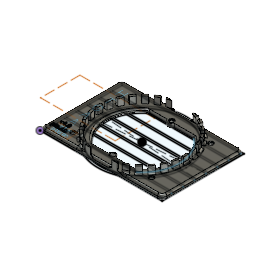
petriDishHolderRibsAndClaw (Autodesk Fusion 360 design; units mm, degrees)
Autodesk Fusion 360 part; units mm, degrees
sketch "main" plane through (0, 0, 0) normal (0, 0, 1) x (1, 0, 0)
  line L0 (0, 0) -> (127.76, 0)
  line L1 (127.76, 0) -> (127.76, 85.57)
  line L2 (127.76, 85.57) -> (0, 85.57)
  line L3 (0, 85.57) -> (0, 0)
  circle A0 centre (63.88, 42.785) radius 43.6
  circle A1 centre (63.88, 42.785) radius 46.2
  line L4 (-29.3174, 29.9498) -> (48.6581, 29.9498) construction
  line L5 (48.6581, 29.9498) -> (48.6581, 71.0126) construction
  line L6 (48.6581, 71.0126) -> (-29.3174, 71.0126) construction
  line L7 (-29.3174, 71.0126) -> (-29.3174, 29.9498) construction
  line L8 (2, 6.3389) -> (22.2506, 6.3389) construction
  line L9 (22.2506, 6.3389) -> (22.2506, 17.2311) construction
  line L10 (22.2506, 17.2311) -> (2, 17.2311) construction
  line L11 (2, 17.2311) -> (2, 6.3389) construction
  line L12 (41.8836, 72.785) -> (88.3277, 72.785)
  line L13 (41.8836, 12.785) -> (88.3277, 12.785)
  arc A2 (41.8836, 72.785) -> (41.8836, 12.785) centre (63.88, 42.785) ccw
  arc A3 (88.3277, 12.785) -> (88.3277, 72.785) centre (63.88, 42.785) ccw
  circle A4 centre (63.88, 42.785) radius 43.2
  line L14 (2, 47.785) -> (125.7601, 47.785)
  line L15 (125.76, 47.785) -> (125.76, 37.785)
  line L16 (125.76, 37.785) -> (2, 37.785)
  line L17 (2, 37.785) -> (2, 47.785)
  line L18 (2, 47.785) -> (125.76, 37.785) construction
  line L19 (125.76, 47.785) -> (2, 37.785) construction
  line L20 (125.7601, 47.785) -> (125.76, 47.785)
  line L21 (2, 11.785) -> (125.7601, 11.785)
  line L22 (2, 1.785) -> (2, 11.785)
  line L23 (125.76, 1.785) -> (2, 1.785)
  line L24 (125.76, 11.785) -> (125.76, 1.785)
  line L25 (125.7601, 11.785) -> (125.76, 11.785)
  line L26 (2, 23.785) -> (125.7601, 23.785)
  line L27 (2, 13.785) -> (2, 23.785)
  line L28 (125.76, 13.785) -> (2, 13.785)
  line L29 (125.76, 23.785) -> (125.76, 13.785)
  line L30 (125.7601, 23.785) -> (125.76, 23.785)
  line L31 (2, 35.785) -> (125.7601, 35.785)
  line L32 (2, 25.785) -> (2, 35.785)
  line L33 (125.76, 25.785) -> (2, 25.785)
  line L34 (125.76, 35.785) -> (125.76, 25.785)
  line L35 (125.7601, 35.785) -> (125.76, 35.785)
  line L36 (2, 59.785) -> (125.7601, 59.785)
  line L37 (2, 49.785) -> (2, 59.785)
  line L38 (125.76, 49.785) -> (2, 49.785)
  line L39 (125.76, 59.785) -> (125.76, 49.785)
  line L40 (125.7601, 59.785) -> (125.76, 59.785)
  line L41 (2, 71.785) -> (125.7601, 71.785)
  line L42 (2, 61.785) -> (2, 71.785)
  line L43 (125.76, 61.785) -> (2, 61.785)
  line L44 (125.76, 71.785) -> (125.76, 61.785)
  line L45 (125.7601, 71.785) -> (125.76, 71.785)
  line L46 (2, 83.785) -> (125.7601, 83.785)
  line L47 (2, 73.785) -> (2, 83.785)
  line L48 (125.76, 73.785) -> (2, 73.785)
  line L49 (125.76, 83.785) -> (125.76, 73.785)
  line L50 (125.7601, 83.785) -> (125.76, 83.785)
  point P0 (63.88, 42.785)
  dimension "d4" = 127.76
  dimension "d5" = 85.57
  dimension "d6" = 87.2
  dimension "d10" = 63.88
  dimension "d11" = 42.785
  dimension "d12" = 92.4
  dimension "d39" = 74.4
  dimension "d42" = 8
  dimension "d61" = 4
  dimension "d67" = 30
  dimension "d68" = 30
  dimension "d72" = 86.4
  dimension "d78" = 10
  dimension "d81" = 0
  dimension "d82" = 12
  dimension "d86" = 2
  dimension "d87" = 5
  text T0 "v1.6\nplastic" font "Arial" height 4 align centre middle in box 20.2506 x 10.8923 at (2, 6.3389) x (1, 0) y (0, 1) spacing 1 kerned
  constraint horizontal L0
  constraint vertical L1
  constraint horizontal L2
  constraint vertical L3
  constraint coincident L0.start L3.end
  constraint concentric A0 A1
  constraint concentric A0 A2
  constraint horizontal L12
  constraint horizontal L13
  constraint concentric A2 A3
  constraint coincident L12.end A3.end
  constraint coincident L12.start A2.start
  constraint concentric A3 A4
  constraint horizontal L14
  constraint perpendicular L14 L15
  constraint parallel L14 L16
  constraint parallel L15 L17
  constraint coincident L18 P0
  constraint coincident L19 P0
  constraint coincident P0 A0.centre
  constraint coincident L21.start
  constraint coincident L21
  measures "d4" distance of L0.start L0.end
  measures "d5" distance of L0.start L2.end
  measures "d6" diameter of A0
  measures "d10" horizontal distance of L0.start A0.centre
  measures "d11" vertical distance of L0.start A0.centre
  measures "d12" diameter of A1
  measures "d39" diameter of A2
  measures "d67" distance of P0 L12
  measures "d68" distance of P0 L13
  measures "d72" diameter of A4
  measures "d78" distance of L14.start L16.end
  measures "d86" distance of L1 L15
  measures "d87" distance of P0 L14
extrude "Extrude1" add sketch "main" along normal blind 4 contours L0 L2 L3 A1 L14 L16 L17 L21 L22 L23 L26 L27 L28 L31 L32 L33 L36 L37 L38 L41 L42 L43 L46 L47 L48 | L0 A0 A1 L23 | L0 A0 A4 L23 | A1 L21 L22 L23 | A0 A1 L21 L23 | L0 L1 L2 A1 L14 L15 L16 L21 L23 L24 L26 L28 L29 L31 L33 L34 L36 L38 L39 L41 L43 L44 L46 L48 L49 | L0 A0 A1 L23 | L2 A0 A1 L46 | L0 A4 L23 | A0 A4 L21 L23 | L0 A0 A4 L23 | A0 A1 L21 L28 | A0 A1 L21 L23 | A1 L21 L23 L24 | L2 A0 A4 L46 | L2 A0 A1 L46 | A0 A1 L46 L48 | A1 L46 L47 L48 | A4 L21 L23 | A0 A4 L21 L28 | A0 A4 L21 L23 | A1 L26 L27 L28 | A0 A1 L26 L28 | A0 A1 L21 L28 | L2 A4 L46 | L2 A0 A4 L46 | A0 A4 L46 L48 | A1 L46 L48 L49 | A0 A1 L46 L48 | A0 A1 L41 L48 | L13 A2 A3 A4 L21 L28 | A0 A4 L26 L28 | A0 A4 L21 L28 | A0 A1 L26 L33 | A0 A1 L26 L28 | A1 L26 L28 L29 | A4 L46 L48 | A0 A4 L46 L48 | A0 A4 L41 L48 | A0 A1 L41 L48 | A0 A1 L41 L43 | A1 L41 L42 L43 | A2 A4 L26 L28 | A0 A4 L26 L33 | A0 A4 L26 L28 | A1 L31 L32 L33 | A0 A1 L31 L33 | A0 A1 L26 L33 | L12 A2 A3 A4 L41 L48 | A0 A4 L41 L48 | A0 A4 L41 L43 | A1 L41 L43 L44 | A0 A1 L41 L43 | A0 A1 L36 L43 | A3 A4 L26 L28 | A2 A4 L26 L33 | L13 A2 A3 L28 | A2 A3 L26 L28 | A0 A4 L31 L33 | A0 A4 L26 L33 | A0 A1 L16 L31 | A0 A1 L31 L33 | A1 L31 L33 L34 | A2 A4 L41 L43 | A0 A4 L41 L43 | A0 A4 L36 L43 | A0 A1 L36 L43 | A0 A1 L36 L38 | A1 L36 L37 L38 | A3 A4 L26 L33 | A2 A4 L31 L33 | A2 A3 L26 L33 | A0 A4 L16 L31 | A0 A4 L31 L33 | A1 L14 L16 L17 | A0 A1 L14 L16 | A0 A1 L16 L31 | A3 A4 L41 L43 | A2 A4 L36 L43 | A2 A3 L41 L43 | L12 A2 A3 L41 | A0 A4 L36 L43 | A0 A4 L36 L38 | A1 L36 L38 L39 | A0 A1 L36 L38 | A0 A1 L14 L38 | A3 A4 L31 L33 | A2 A4 L16 L31 | A2 A3 L31 L33 | A0 A4 L14 L16 | A0 A4 L16 L31 | A0 A1 L14 L16 | A1 L14 L15 L16 | A3 A4 L36 L43 | A2 A4 L36 L38 | A2 A3 L36 L43 | A0 A4 L36 L38 | A0 A4 L14 L38 | A0 A1 L14 L38 | A3 A4 L16 L31 | A2 A4 L14 L16 | A2 A3 L16 L31 | A0 A4 L14 L16 | A3 A4 L36 L38 | A2 A4 L14 L38 | A2 A3 L36 L38 | A0 A4 L14 L38 | A3 A4 L14 L16 | A2 A3 L14 L16 | A3 A4 L14 L38 | A2 A3 L14 L38 makes body 1
extrude "Extrude2" add sketch "main" along normal blind 7 from surface at 4 contours L0 A0 A1 L23 | A0 A1 L21 L23 | L0 A0 A1 L23 | L2 A0 A1 L46 | A0 A1 L21 L28 | A0 A1 L21 L23 | L2 A0 A1 L46 | A0 A1 L46 L48 | A0 A1 L26 L28 | A0 A1 L21 L28 | A0 A1 L46 L48 | A0 A1 L41 L48 | A0 A1 L26 L33 | A0 A1 L26 L28 | A0 A1 L41 L48 | A0 A1 L41 L43 | A0 A1 L31 L33 | A0 A1 L26 L33 | A0 A1 L41 L43 | A0 A1 L36 L43 | A0 A1 L16 L31 | A0 A1 L31 L33 | A0 A1 L36 L43 | A0 A1 L36 L38 | A0 A1 L14 L16 | A0 A1 L16 L31 | A0 A1 L36 L38 | A0 A1 L14 L38 | A0 A1 L14 L16 | A0 A1 L14 L38 bodies 1
extrude "Extrude6" add sketch "main" along normal blind 2 from surface at 9 contours L0 A0 A4 L23 | A0 A4 L21 L23 | L2 A0 A4 L46 | A0 A4 L21 L28 | A0 A4 L46 L48 | A0 A4 L26 L28 | A0 A4 L41 L48 | A0 A4 L26 L33 | A0 A4 L41 L43 | A0 A4 L31 L33 | A0 A4 L36 L43 | A0 A4 L16 L31 | A0 A4 L36 L38 | A0 A4 L14 L16 | A0 A4 L14 L38 picked at (76.3561, 1.3005) picked at (79.8883, 2.6163) picked at (76.3561, 84.2695) picked at (94.3772, 12.0026) picked at (79.8883, 82.9537) picked at (96.9347, 14.824) picked at (94.3772, 73.5674) picked at (102.9314, 24.0055) picked at (96.9347, 70.746) picked at (104.1525, 26.8688) picked at (102.9314, 61.5645) picked at (106.6788, 36.0067) picked at (104.1525, 58.7012) picked at (106.9776, 47.2308) picked at (106.6788, 49.5633) bodies 1
fillet "Fillet9" radius 1 1 edges at (107.08, 42.785, 9) on bodies 1
fillet "Fillet9" radius 1 1 edges at (107.08, 42.785, 11) on bodies 1
fillet "Fillet4" radius 2 2 edges at (17.68, 42.785, 4) (110.08, 42.785, 4) on bodies 1
fillet "Fillet5" radius 2 13 edges at (0, 42.785, 4) (63.88, 85.57, 4) (106.9182, 85.57, 4) (83.3417, 85.57, 4.3962) (81.3123, 85.57, 8.5) (127.76, 42.785, 4) (81.3123, 0, 8.5) (83.3417, 0, 4.3962) (106.9182, 0, 4) (63.88, 0, 4) (20.8418, 0, 4) (44.4183, 0, 4.3962) (46.4477, 0, 8.5) on bodies 1
fillet "Fillet5" radius 2 3 edges at (46.4477, 85.57, 8.5) (44.4183, 85.57, 4.3962) (20.8418, 85.57, 4) on bodies 1
fillet "corners" radius 5 2 edges at (0, 0, 1) (0.5858, 0.5858, 3.4142) on bodies 1
fillet "corners" radius 5 2 edges at (127.76, 85.57, 1) (127.1742, 84.9842, 3.4142) on bodies 1
fillet "corners" radius 5 2 edges at (0.5858, 84.9842, 3.4142) (0, 85.57, 1) on bodies 1
fillet "corners" radius 5 2 edges at (127.76, 0, 1) (127.1742, 0.5858, 3.4142) on bodies 1
extrude "Extrude3" cut sketch "main" along normal blind 4 contours L13 A2 A3 L28 | A2 A3 L26 L28 | A2 A3 L26 L33 | A2 A3 L41 L43 | L12 A2 A3 L41 | A2 A3 L31 L33 | A2 A3 L36 L43 | A2 A3 L16 L31 | A2 A3 L36 L38 | A2 A3 L14 L16 | A2 A3 L14 L38 bodies 1
extrude "Extrude5" add sketch "main" along normal blind 1 from surface at 4 text T0 bodies 1
chamfer "Chamfer3" distance 1.5 angle 45 3 edges at (26.68, 42.785, 4) (102.58, 42.785, 4) (65.1057, 12.785, 4) tangent chain off on bodies 1
extrude "Extrude7" cut sketch "main" along normal blind 1 contours A1 L21 L22 L23 | A0 A1 L21 L23 | A0 A4 L21 L23 | A0 A1 L21 L23 | A1 L21 L23 L24 | L2 A0 A4 L46 | A0 A1 L46 L48 | A1 L46 L47 L48 | A4 L21 L23 | A0 A4 L21 L23 | A1 L26 L27 L28 | A0 A1 L26 L28 | L2 A0 A4 L46 | A0 A4 L46 L48 | A1 L46 L48 L49 | A0 A1 L46 L48 | A0 A1 L41 L48 | A0 A4 L26 L28 | A0 A1 L26 L33 | A0 A1 L26 L28 | A1 L26 L28 L29 | A4 L46 L48 | A0 A4 L46 L48 | A0 A1 L41 L48 | A0 A1 L41 L43 | A1 L41 L42 L43 | A2 A4 L26 L28 | A0 A4 L26 L28 | A1 L31 L32 L33 | A0 A1 L31 L33 | A0 A1 L26 L33 | A1 L41 L43 L44 | A0 A1 L41 L43 | A0 A1 L36 L43 | A3 A4 L26 L28 | A2 A3 L26 L28 | A0 A4 L31 L33 | A0 A1 L16 L31 | A0 A1 L31 L33 | A1 L31 L33 L34 | A2 A4 L41 L43 | A0 A1 L36 L43 | A0 A1 L36 L38 | A1 L36 L37 L38 | A2 A4 L31 L33 | A0 A4 L31 L33 | A1 L14 L16 L17 | A0 A1 L14 L16 | A0 A1 L16 L31 | A0 A4 L36 L38 | A1 L36 L38 L39 | A0 A1 L36 L38 | A0 A1 L14 L38 | A3 A4 L31 L33 | A2 A3 L31 L33 | A0 A4 L14 L16 | A0 A1 L14 L16 | A1 L14 L15 L16 | A2 A4 L36 L38 | A0 A4 L36 L38 | A0 A1 L14 L38 | A2 A4 L14 L16 | A0 A4 L14 L16 | A3 A4 L36 L38 | A2 A3 L36 L38 | A3 A4 L14 L16 | A2 A3 L14 L16 bodies 1
sketch "fingers" plane through (0, 0, 0) normal (0, 0, 1) x (1, 0, 0)
  line L0 (65.88, -8.3696) -> (61.88, -8.3696)
  line L1 (61.88, -8.3696) -> (61.88, 93.9396)
  line L2 (61.88, 93.9396) -> (65.88, 93.9396)
  line L3 (65.88, 93.9396) -> (65.88, -8.3696)
  line L4 (65.88, -8.3696) -> (61.88, 93.9396) construction
  line L5 (61.88, -8.3696) -> (65.88, 93.9396) construction
  line L6 (61.88, -8.3696) -> (61.88, 93.9396)
  line L7 (65.88, -8.3696) -> (61.88, -8.3696)
  line L8 (65.88, 93.9396) -> (65.88, -8.3696)
  line L9 (61.88, 93.9396) -> (65.88, 93.9396)
  line L10 (51.2881, 92.4059) -> (55.2007, 93.2376)
  line L11 (55.2007, 93.2376) -> (76.4719, -6.8359)
  line L12 (72.5593, -7.6676) -> (51.2881, 92.4059)
  line L13 (76.4719, -6.8359) -> (72.5593, -7.6676)
  line L14 (41.2465, 88.7036) -> (44.9006, 90.3305)
  line L15 (44.9006, 90.3305) -> (86.5135, -3.1336)
  line L16 (82.8594, -4.7605) -> (41.2465, 88.7036)
  line L17 (86.5135, -3.1336) -> (82.8594, -4.7605)
  line L18 (32.194, 82.9944) -> (35.4301, 85.3455)
  line L19 (35.4301, 85.3455) -> (95.566, 2.5756)
  line L20 (92.3299, 0.2245) -> (32.194, 82.9944)
  line L21 (95.566, 2.5756) -> (92.3299, 0.2245)
  line L22 (24.5265, 75.5278) -> (27.203, 78.5004)
  line L23 (27.203, 78.5004) -> (103.2335, 10.0422)
  line L24 (100.557, 7.0696) -> (24.5265, 75.5278)
  line L25 (103.2335, 10.0422) -> (100.557, 7.0696)
  line L26 (18.5788, 66.6303) -> (20.5788, 70.0944)
  line L27 (20.5788, 70.0944) -> (109.1812, 18.9397)
  line L28 (107.1812, 15.4756) -> (18.5788, 66.6303)
  line L29 (109.1812, 18.9397) -> (107.1812, 15.4756)
  line L30 (14.611, 56.6905) -> (15.8471, 60.4948)
  line L31 (15.8471, 60.4948) -> (113.149, 28.8795)
  line L32 (111.9129, 25.0752) -> (14.611, 56.6905)
  line L33 (113.149, 28.8795) -> (111.9129, 25.0752)
  line L34 (12.7966, 46.1431) -> (13.2147, 50.1212)
  line L35 (13.2147, 50.1212) -> (114.9634, 39.4269)
  line L36 (114.5453, 35.4488) -> (12.7966, 46.1431)
  line L37 (114.9634, 39.4269) -> (114.5453, 35.4488)
  line L38 (13.2147, 35.4488) -> (12.7966, 39.4269)
  line L39 (12.7966, 39.4269) -> (114.5453, 50.1212)
  line L40 (114.9634, 46.1431) -> (13.2147, 35.4488)
  line L41 (114.5453, 50.1212) -> (114.9634, 46.1431)
  line L42 (15.8471, 25.0752) -> (14.611, 28.8795)
  line L43 (14.611, 28.8795) -> (111.9129, 60.4948)
  line L44 (113.149, 56.6905) -> (15.8471, 25.0752)
  line L45 (111.9129, 60.4948) -> (113.149, 56.6905)
  line L46 (20.5788, 15.4756) -> (18.5788, 18.9397)
  line L47 (18.5788, 18.9397) -> (107.1812, 70.0944)
  line L48 (109.1812, 66.6303) -> (20.5788, 15.4756)
  line L49 (107.1812, 70.0944) -> (109.1812, 66.6303)
  line L50 (27.203, 7.0696) -> (24.5265, 10.0422)
  line L51 (24.5265, 10.0422) -> (100.557, 78.5004)
  line L52 (103.2335, 75.5278) -> (27.203, 7.0696)
  line L53 (100.557, 78.5004) -> (103.2335, 75.5278)
  line L54 (35.4301, 0.2245) -> (32.194, 2.5756)
  line L55 (32.194, 2.5756) -> (92.3299, 85.3455)
  line L56 (95.566, 82.9944) -> (35.4301, 0.2245)
  line L57 (92.3299, 85.3455) -> (95.566, 82.9944)
  line L58 (44.9006, -4.7605) -> (41.2465, -3.1336)
  line L59 (41.2465, -3.1336) -> (82.8594, 90.3305)
  line L60 (86.5135, 88.7036) -> (44.9006, -4.7605)
  line L61 (82.8594, 90.3305) -> (86.5135, 88.7036)
  line L62 (55.2007, -7.6676) -> (51.2881, -6.8359)
  line L63 (51.2881, -6.8359) -> (72.5593, 93.2376)
  line L64 (76.4719, 92.4059) -> (55.2007, -7.6676)
  line L65 (72.5593, 93.2376) -> (76.4719, 92.4059)
  line L66 (65.88, -8.3696) -> (61.88, -8.3696)
  line L67 (61.88, -8.3696) -> (61.88, 93.9396)
  line L68 (65.88, 93.9396) -> (65.88, -8.3696)
  line L69 (61.88, 93.9396) -> (65.88, 93.9396)
  line L70 (76.4719, -6.8359) -> (72.5593, -7.6676)
  line L71 (72.5593, -7.6676) -> (51.2881, 92.4059)
  line L72 (55.2007, 93.2376) -> (76.4719, -6.8359)
  line L73 (51.2881, 92.4059) -> (55.2007, 93.2376)
  line L74 (86.5135, -3.1336) -> (82.8594, -4.7605)
  line L75 (82.8594, -4.7605) -> (41.2465, 88.7036)
  line L76 (44.9006, 90.3305) -> (86.5135, -3.1336)
  line L77 (41.2465, 88.7036) -> (44.9006, 90.3305)
  line L78 (95.566, 2.5756) -> (92.3299, 0.2245)
  line L79 (92.3299, 0.2245) -> (32.194, 82.9944)
  line L80 (35.4301, 85.3455) -> (95.566, 2.5756)
  line L81 (32.194, 82.9944) -> (35.4301, 85.3455)
  line L82 (103.2335, 10.0422) -> (100.557, 7.0696)
  line L83 (100.557, 7.0696) -> (24.5265, 75.5278)
  line L84 (27.203, 78.5004) -> (103.2335, 10.0422)
  line L85 (24.5265, 75.5278) -> (27.203, 78.5004)
  line L86 (109.1812, 18.9397) -> (107.1812, 15.4756)
  line L87 (107.1812, 15.4756) -> (18.5788, 66.6303)
  line L88 (20.5788, 70.0944) -> (109.1812, 18.9397)
  line L89 (18.5788, 66.6303) -> (20.5788, 70.0944)
  line L90 (113.149, 28.8795) -> (111.9129, 25.0752)
  line L91 (111.9129, 25.0752) -> (14.611, 56.6905)
  line L92 (15.8471, 60.4948) -> (113.149, 28.8795)
  line L93 (14.611, 56.6905) -> (15.8471, 60.4948)
  line L94 (114.9634, 39.4269) -> (114.5453, 35.4488)
  line L95 (114.5453, 35.4488) -> (12.7966, 46.1431)
  line L96 (13.2147, 50.1212) -> (114.9634, 39.4269)
  line L97 (12.7966, 46.1431) -> (13.2147, 50.1212)
  line L98 (114.5453, 50.1212) -> (114.9634, 46.1431)
  line L99 (114.9634, 46.1431) -> (13.2147, 35.4488)
  line L100 (12.7966, 39.4269) -> (114.5453, 50.1212)
  line L101 (13.2147, 35.4488) -> (12.7966, 39.4269)
  line L102 (111.9129, 60.4948) -> (113.149, 56.6905)
  line L103 (113.149, 56.6905) -> (15.8471, 25.0752)
  line L104 (14.611, 28.8795) -> (111.9129, 60.4948)
  line L105 (15.8471, 25.0752) -> (14.611, 28.8795)
  line L106 (107.1812, 70.0944) -> (109.1812, 66.6303)
  line L107 (109.1812, 66.6303) -> (20.5788, 15.4756)
  line L108 (18.5788, 18.9397) -> (107.1812, 70.0944)
  line L109 (20.5788, 15.4756) -> (18.5788, 18.9397)
  line L110 (100.557, 78.5004) -> (103.2335, 75.5278)
  line L111 (103.2335, 75.5278) -> (27.203, 7.0696)
  line L112 (24.5265, 10.0422) -> (100.557, 78.5004)
  line L113 (27.203, 7.0696) -> (24.5265, 10.0422)
  line L114 (92.3299, 85.3455) -> (95.566, 82.9944)
  line L115 (95.566, 82.9944) -> (35.4301, 0.2245)
  line L116 (32.194, 2.5756) -> (92.3299, 85.3455)
  line L117 (35.4301, 0.2245) -> (32.194, 2.5756)
  line L118 (82.8594, 90.3305) -> (86.5135, 88.7036)
  line L119 (86.5135, 88.7036) -> (44.9006, -4.7605)
  line L120 (41.2465, -3.1336) -> (82.8594, 90.3305)
  line L121 (44.9006, -4.7605) -> (41.2465, -3.1336)
  line L122 (72.5593, 93.2376) -> (76.4719, 92.4059)
  line L123 (76.4719, 92.4059) -> (55.2007, -7.6676)
  line L124 (51.2881, -6.8359) -> (72.5593, 93.2376)
  line L125 (55.2007, -7.6676) -> (51.2881, -6.8359)
  line L126 (56.38, 102.785) -> (71.38, 102.785)
  line L127 (71.38, 102.785) -> (71.38, -17.215)
  line L128 (71.38, -17.215) -> (56.38, -17.215)
  line L129 (56.38, -17.215) -> (56.38, 102.785)
  line L130 (56.38, 102.785) -> (71.38, -17.215) construction
  line L131 (71.38, 102.785) -> (56.38, -17.215) construction
  point P0 (63.88, 42.785)
  point P1 (63.88, 42.785)
  point P2 (63.88, 42.785)
  dimension "d88" = 4
  dimension "d90" = 360
  dimension "d95" = 360
  dimension "d99" = 120
  dimension "d100" = 15
  constraint horizontal L0
  constraint perpendicular L0 L1
  constraint parallel L0 L2
  constraint parallel L1 L3
  constraint coincident L4 P2
  constraint coincident L5 P2
  constraint coincident P2 P1
  constraint horizontal L126
  constraint perpendicular L126 L127
  constraint parallel L126 L128
  constraint parallel L127 L129
  constraint coincident L130 P2
  constraint coincident L131 P2
  measures "d88" distance of L1.end L2.end
  measures "d99" distance of L126.end L127.end
  measures "d100" distance of L126.start L126.end
extrude "Extrude9" cut sketch "fingers" along normal blind 15 from surface at 4 contours L0 L1 L3 L6 L7 L8 L12 L64 L66 L67 L68 L71 L123 | L3 L8 L11 L12 L16 L68 L71 L72 L75 L127 | L1 L6 L60 L63 L64 L67 L119 L123 L124 L129 | L11 L12 L13 L70 L71 L72 L127 | L62 L63 L64 L123 L124 L125 L129 | L11 L16 L20 L72 L75 L79 L127 | L56 L60 L63 L115 L119 L124 L129 | L15 L16 L17 L20 L74 L75 L76 L79 L127 | L56 L58 L59 L60 L115 L119 L120 L121 L129 | L15 L24 L76 L83 L127 | L15 L19 L20 L21 L24 L76 L78 L79 L80 L83 L127 | L52 L59 L111 L120 L129 | L52 L54 L55 L56 L59 L111 L115 L116 L117 L120 L129 | L19 L28 L80 L87 L127 | L19 L23 L24 L25 L28 L80 L82 L83 L84 L87 L127 | L48 L55 L107 L116 L129 | L48 L50 L51 L52 L55 L107 L111 L112 L113 L116 L129 | L23 L27 L28 L29 L32 L84 L86 L87 L88 L91 | L44 L46 L47 L48 L51 L103 L107 L108 L109 L112 | L27 L31 L32 L33 L36 L88 L90 L91 L92 L95 | L40 L42 L43 L44 L47 L99 L103 L104 L105 L108 | L31 L35 L36 L37 L40 L92 L94 L95 L96 L99 | L36 L38 L39 L40 L43 L95 L99 L100 L101 L104 | L35 L39 L40 L41 L44 L96 L98 L99 L100 L103 | L32 L34 L35 L36 L39 L91 L95 L96 L97 L100 | L39 L43 L44 L45 L48 L100 L102 L103 L104 L107 | L28 L30 L31 L32 L35 L87 L91 L92 L93 L96 | L43 L47 L48 L49 L52 L104 L106 L107 L108 L111 | L24 L26 L27 L28 L31 L83 L87 L88 L89 L92 | L47 L56 L108 L115 L127 | L47 L51 L52 L53 L56 L108 L110 L111 L112 L115 L127 | L20 L27 L79 L88 L129 | L20 L22 L23 L24 L27 L79 L83 L84 L85 L88 L129 | L51 L60 L112 L119 L127 | L51 L55 L56 L57 L60 L112 L114 L115 L116 L119 L127 | L16 L23 L75 L84 L129 | L16 L18 L19 L20 L23 L75 L79 L80 L81 L84 L129 | L55 L59 L64 L116 L120 L123 L127 | L55 L59 L60 L61 L116 L118 L119 L120 L127 | L12 L15 L19 L71 L76 L80 L129 | L14 L15 L16 L19 L75 L76 L77 L80 L129 | L3 L8 L59 L63 L64 L68 L120 L123 L124 L127 | L1 L6 L11 L12 L15 L67 L71 L72 L76 L129 | L1 L2 L3 L6 L8 L9 L11 L63 L67 L68 L69 L72 L124 | L63 L64 L65 L122 L123 L124 L127 | L10 L11 L12 L71 L72 L73 L129 bodies 1 makes body 2 at (70.772, 0, 9.7303) makes body 3 at (70.772, 85.57, 9.7303)
extrude "Extrude10" cut sketch "fingers" along normal blind 7 from surface at 4 contours L0 L1 L3 L6 L7 L8 L12 L64 L66 L67 L68 L71 L123 L127 L128 L129 | L1 L2 L3 L6 L8 L9 L11 L63 L67 L68 L69 L72 L124 L126 L127 L129 bodies 3 2 1
sketch "screws" plane through (0, 0, 0) normal (0, 0, 1) x (1, 0, 0)
  circle A0 centre (22.88, 73.935) radius 2.65
  circle A1 centre (22.88, 11.635) radius 1.8
  circle A2 centre (22.88, 73.935) radius 3.8
  circle A3 centre (63.88, 73.935) radius 2.65
  circle A4 centre (22.88, 11.635) radius 3.8
  circle A5 centre (63.88, 11.635) radius 2.65
  circle A6 centre (63.88, 73.935) radius 3.8
  circle A7 centre (63.88, 11.635) radius 3.8
  circle A8 centre (63.88, 73.935) radius 1.8
  circle A9 centre (63.88, 11.635) radius 1.8
  circle A10 centre (22.88, 11.635) radius 2.65
  circle A11 centre (22.88, 73.935) radius 1.8
  circle A12 centre (104.88, 73.935) radius 1.8
  circle A13 centre (104.88, 73.935) radius 3.8
  circle A14 centre (104.88, 73.935) radius 2.65
  circle A15 centre (104.88, 11.635) radius 1.8
  circle A16 centre (104.88, 11.635) radius 3.8
  circle A17 centre (104.88, 11.635) radius 2.65
  point P0 (63.88, 42.785)
  point P1 (63.88, 42.785)
  dimension "d122" = 41
  dimension "d124" = 3.6
  dimension "d125" = 41
  dimension "d126" = 31.15
  dimension "d127" = 7.6
  dimension "d128" = 5.3
  constraint concentric A2 A11
  constraint concentric A0 A11
  constraint coincident P1 P0
  measures "d124" diameter of A11
  measures "d125" horizontal distance of A0.centre P1
  measures "d126" vertical distance of A3.centre P1
  measures "d127" diameter of A2
  measures "d128" diameter of A0
extrude "Extrude14" cut sketch "screws" along normal blind 4 contours A1 | A8 | A9 | A11 | A12 | A15 bodies 1
extrude "Extrude15" cut sketch "screws" along normal blind 1 from surface at 3 contours A0 | A3 | A5 | A10 | A14 | A17 bodies 1
extrude "Extrude16" add sketch "screws" along normal blind 4 contours A2 | A4 | A6 | A7 bodies 2 3 1
extrude "Extrude4" [rolled back] along distance 1 taper angle 0 profile offset 4
sketch "testOnly" plane through (0, 0, 0) normal (0, 0, 1) x (1, 0, 0)
  circle A0 centre (63.7141, 42.9318) radius 45.3838
  line L0 (-3.7661, 109.9971) -> (141.9216, 109.9971)
  line L1 (141.9216, 109.9971) -> (141.9216, -22.287)
  line L2 (141.9216, -22.287) -> (-3.7661, -22.287)
  line L3 (-3.7661, -22.287) -> (-3.7661, 109.9971)
  circle A1 centre (63.7141, 42.9318) radius 40.8847
  constraint horizontal L0
  constraint vertical L1
  constraint horizontal L2
  constraint vertical L3
  constraint concentric A0 A1
extrude "Extrude11" [rolled back] along distance 10 taper angle 0
extrude "Extrude12" [rolled back] along distance 2.5 taper angle 0
extrude "Extrude13" [rolled back] along distance 10 taper angle 0
equation "length = 127.76 mm" comment "127.5"
equation "width = 85.57 mm" comment "85.5"
equation "totalHeight = 11 mm"
equation "d4 = length"
equation "d5 = width"
equation "d6 = petriHoleDiameter"
equation "petriMeasuredDiameter = 86.4 mm"
equation "petriWall = 3 mm"
equation "baseHeight = 4 mm"
equation "d10 = length / 2"
equation "d11 = width / 2"
equation "d12 = petriMeasuredDiameter + 2 * petriWall"
equation "d13 = baseHeight"
equation "d15 = totalHeight - baseHeight"
equation "d20 = baseHeight"
equation "d39 = petriMeasuredDiameter - 12 mm"
equation "d40 = baseHeight"
equation "d45 = baseHeight"
equation "d62 = baseHeight"
equation "d72 = petriHoleDiameter - clawDepth"
equation "d73 = totalHeight - 2 mm"
equation "d96 = baseHeight"
equation "d97 = totalHeight - -baseHeight"
equation "d101 = baseHeight"
equation "d102 = totalHeight - baseHeight"
equation "petriHoleDiameter = petriMeasuredDiameter + play"
equation "play = 0.8 mm"
equation "clawDepth = 0.8 mm"
equation "screwDiameterIncludingPlay = 3.2 mm"
equation "screwHeadDiameter = 6.2 mm"
equation "screwXDistanceX = 82 mm"
equation "d122 = screwXDistanceX / 2"
equation "d123 = -screwYDistanceX"
equation "d125 = screwXDistanceX / 2"
equation "d129 = baseHeight"
equation "d131 = baseHeight - 1 mm"
equation "d134 = baseHeight"
equation "screwYDistanceX = 62.30 mm"
named bodies: "petri holder with claws", "petri holder with claws (1)", "petri holder with claws (2)"
